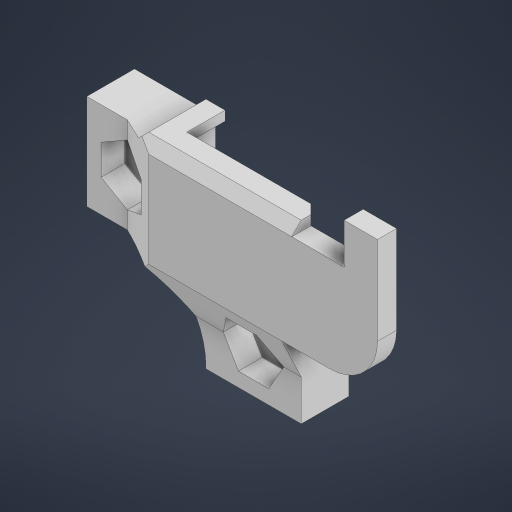
# Autodesk Inventor part: motor_clamp_L_nutt_left1
Saved by Autodesk Inventor 2024 (Build 280153000, 153)
## iProperties
Created: 2024-04-12
Part Number: motor_clamp_L_nutt_left1
Material: Všeobecné
Document SubType Name: Modeling
Designer: Simak
Density: 1 g/cm^3
Appearance: Výchozí
Author: Simak
Autodesk Inventor part; units mm, degrees
ref_plane "YZ Plane" through (0, 0, 0) normal (1, 0, 0) x (0, 1, 0)
ref_plane "XZ Plane" through (0, 0, 0) normal (0, 1, 0) x (-1, 0, 0)
ref_plane "XY Plane" through (0, 0, 0) normal (0, 0, 1) x (1, 0, 0)
sketch "Náčrt1" plane through (0, 0, 0) normal (0, 0, 1) x (1, 0, 0)
  line L0 (-13.5, 5) -> (-13.5, -5)
  line L1 (-13.5, -5) -> (-5, -5)
  line L2 (-5, -5) -> (-5, 5)
  line L3 (-5, 5) -> (-13.5, 5)
  line L4 (-5, -5) -> (14, -5)
  arc A0 (14, -5) -> (14, 5) centre (14, 0) ccw
  line L5 (14, 5) -> (-5, 5)
  line L6 (-1, 5) -> (-1, 13.5)
  line L7 (-1, 13.5) -> (9, 13.5)
  line L8 (9, 13.5) -> (9, 5)
  line L9 (-5, -5) -> (0, 0) construction
  line L10 (0, 0) -> (-5, 5) construction
  line L11 (-13.5, 5) -> (-9.25, 0) construction
  line L12 (-9.25, 0) -> (-5, 5) construction
  line L13 (-9.25, 0) -> (-13.5, -5) construction
  line L14 (-1, 13.5) -> (4, 9.25) construction
  line L15 (4, 9.25) -> (-1, 5) construction
  arc A1 (-9.25, 5) -> (-1, 13.25) centre (-9.25, 13.25) ccw
  circle A2 centre (-9.25, 0) radius 1.65
  circle A3 centre (4, 9.25) radius 1.65
  line L16 (14, -5) -> (19, -5)
  line L17 (19, -5) -> (19, 0)
  dimension "d3" = 24
  dimension "d4" = 8.5
  dimension "d5" = 10
  dimension "d6" = 12.5
  dimension "d40" = 3.3
  constraints: 36 end point, 7 equal length, 7 perpendicular, 5 point on circle, 5 point on line, 5 tangent, 4 centre point, 3 coincident, 2 midpoint, 2 vertical, 1 equal radius, 1 horizontal, 1 parallel, 1 vertical alignment
  measures "d3" distance from line of L17.end L2
  measures "d4" distance between parallel lines of L0 L2
  measures "d5" distance of L0.start L0.end
  measures "d6" distance between parallel lines of L6 L0
  measures "d40" diameter of A2
extrude "Vysunutí1" add sketch "Náčrt1" against normal blind 5 contours L3 L2 L1 L0 | A1 L6 L5 L3 | L6 L7 L8 L5 | A2 | A3
extrude "Vysunutí2" add sketch "Náčrt1" along normal blind 2 contours L2 L5 A0 L4 | A0 L17 L16
sketch "Náčrt2" plane through (-13.5, -5, -5) normal (0, -1, 0) x (1, 0, 0)
  line L0 (27.5, 7) -> (8.5, 7) projected
  line L1 (8.5, 7) -> (4.25, 5)
  line L2 (0, 5) -> (8.5, 5) projected
  line L3 (8.5, 5) -> (27.5, 5) projected
  line L4 (27.5, 5) -> (27.5, 7) projected
  line L5 (8.5, 7) -> (27.5, 7) projected
  line L6 (8.5, 5) -> (8.5, 7) projected
  point P0 (13.5, 5)
  constraints: 2 end point, 1 midpoint
extrude "Vysunutí3" add sketch "Náčrt2" against normal up to surface (10 mm away) contours L6 L2 L1
sketch "Náčrt3" plane through (9, 5, -5) normal (1, 0, 0) x (0, 0, -1)
  line L0 (-5, -5) -> (-5, 0) projected
  line L1 (-5, 0) -> (-7, 0) projected
  line L2 (-7, -5) -> (-7, 0) projected
  line L3 (-5, 0) -> (-5, 8.5) projected
  line L4 (-5, 0) -> (0, 0) projected
  line L5 (0, 8.5) -> (0, 0) projected
  line L6 (-5, 8.5) -> (0, 8.5) projected
  line L7 (-7, 0) -> (-5, 4.25)
  line L8 (-5, -5) -> (-7, -5) projected
  constraints: 2 end point, 1 midpoint
extrude "Vysunutí4" add sketch "Náčrt3" against normal up to surface contours L1 L7 L3 surface through (-9.25, -5, 0) normal (-0.425797, 0, 0.9048187)
sketch "Náčrt4" plane through (-2.0346, 9.25, 0) normal (0, 0, -1) x (-1, 0, 0)
  arc A0 (0, 0) -> (7.2154, -4.25) centre (7.2154, 4) ccw projected
  line L0 (7.2154, -4.25) -> (7.2154, 0) projected
  line L1 (0, 0) -> (7.2154, 0) projected
  point P0 (-2.0346, -9.25)
extrude "Vysunutí5" cut sketch "Náčrt4" against normal through all
sketch "Náčrt6" plane through (-13.5, -5, -5) normal (0, -1, 0) x (1, 0, 0)
  line L0 (8.5, 5) -> (22.5, 5) projected
  line L1 (8.5, 5) -> (8.5, 0) projected
  line L2 (22.5, 0) -> (8.5, 0) projected
  line L3 (22.5, 5) -> (22.5, 0) projected
  line L4 (0, 5) -> (4.25, 5) projected
  line L5 (0, 5) -> (0, 0) projected
  line L6 (8.5, 0) -> (0, 0) projected
  line L7 (8.5, 5) -> (8.5, 0) projected
  line L8 (8.5, 7) -> (4.25, 5) projected
  line L9 (7.5, -1) -> (7.5, 6)
  line L10 (7.5, 6) -> (23.5, 6)
  line L11 (23.5, 6) -> (23.5, -1)
  line L12 (23.5, -1) -> (7.5, -1)
  line L13 (21.5, 4) -> (9.5, 4)
  line L14 (9.5, 4) -> (9.5, 1)
  line L15 (9.5, 1) -> (21.5, 1)
  line L16 (21.5, 1) -> (21.5, 4)
  line L17 (9.5, 1) -> (9.5, 0)
  line L18 (21.5, 4) -> (22.5, 4)
  line L19 (22.5, 4) -> (23.5, 4)
  line L20 (8.5, 5) -> (32.5, 5) projected
  line L21 (32.5, 5) -> (32.5, 7) projected
  line L22 (8.5, 7) -> (32.5, 7) projected
  point P0 (13.5, 5)
  point P1 (7.5, 0)
  dimension "d33" = 1
  dimension "d34" = 1
  constraints: 22 end point, 3 point on line, 2 perpendicular, 1 horizontal, 6 other
  measures "d33" distance between parallel lines of L1 L9
  measures "d34" distance between parallel lines of L0 L13
extrude "Vysunutí7" add sketch "Náčrt6" along normal blind 1 contours L1 L6 L9 L10 L11 L20 L0 | L0 L3 L18 L13 L14 L17 L2 L1 | L20 L11 L19 L3
chamfer "Zkosení1" distance 1 angle 45 3 edges at (10, -5.5, -1) (2, -5, 1) (-6, -5, -2)
extrude "Vysunutí8" cut sketch "Náčrt1" against normal through all contours A2 | A3
sketch "Náčrt7" plane through (0, 0, 0) normal (0, 0, 1) x (1, 0, 0)
  circle A0 centre (4, 9.25) radius 1.65 projected
  line L0 (5.5877, 12) -> (7.1754, 9.25)
  line L1 (7.1754, 9.25) -> (5.5877, 6.5)
  line L2 (5.5877, 6.5) -> (2.4123, 6.5)
  line L3 (2.4123, 6.5) -> (0.8246, 9.25)
  line L4 (0.8246, 9.25) -> (2.4123, 12)
  line L5 (2.4123, 12) -> (5.5877, 12)
  circle A1 centre (-9.25, 0) radius 1.65 projected
  line L6 (-9.25, 3.1754) -> (-6.5, 1.5877)
  line L7 (-6.5, 1.5877) -> (-6.5, -1.5877)
  line L8 (-6.5, -1.5877) -> (-9.25, -3.1754)
  line L9 (-9.25, -3.1754) -> (-12, -1.5877)
  line L10 (-12, -1.5877) -> (-12, 1.5877)
  line L11 (-12, 1.5877) -> (-9.25, 3.1754)
  line L12 (-5, 5) -> (-5, -5) projected
  line L13 (9, 5) -> (-5, 5) projected
  point P0 (0, 0)
  dimension "d43" = 5.5
  constraints: 24 end point, 2 coincident, 2 parallel, 1 equal length, 26 other
  measures "d43" distance between parallel lines of L3 L0
extrude "Vysunutí9" cut sketch "Náčrt7" against normal blind 2.5 contours A0 | L0 L1 L2 L3 L4 L5 | A1 | L6 L7 L8 L9 L10 L11
extrude "Vysunutí10" cut sketch "Náčrt7" along normal through all contours A0 | L0 L1 L2 L3 L4 L5 | A1 | L6 L7 L8 L9 L10 L11
sketch "Náčrt8" plane through (0, 0, 0) normal (0, 0, -1) x (-1, 0, 0)
  line L0 (-19, -5) -> (-19, 0) projected
  line L1 (-19, -5) -> (-15.5, -5)
  line L2 (-15.5, -5) -> (-15.5, -9.25)
  line L3 (-15.5, -9.25) -> (-19, -9.25)
  line L4 (-19, -9.25) -> (-19, -5)
  point P0 (0, 0)
  dimension "d48" = 4.25
  dimension "d49" = 3.5
  constraints: 8 end point, 2 parallel, 1 horizontal, 1 perpendicular
  measures "d48" distance of L3.end L0.start
  measures "d49" distance of L2.end L3.end
extrude "Vysunutí11" add sketch "Náčrt8" against normal up to surface (2 mm away)
mirror "Zrcadlit2" about plane through (-1, 13.5, 0) normal (0, 1, 0) remove original yes
